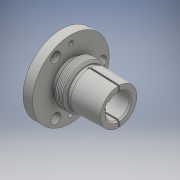
# Autodesk Inventor part: Spannhylsa_2015_HT1
Saved by Autodesk Inventor 2016 (Build 200138000, 138)
## iProperties
Created: 2015-09-08
Part Number: Spannhylsa_2015_HT1
Material: Generic
Document SubType Name: Modeling
Designer: hesaon
Density: 1 g/cm^3
Appearance: Default
Author: hesaon
Title: Spannhylsa_2015_HT1
Autodesk Inventor part; units mm, degrees
ref_plane "YZ Plane" through (0, 0, 0) normal (1, 0, 0) x (0, 1, 0)
ref_plane "XY Plane" through (0, 0, 0) normal (0, 0, 1) x (1, 0, 0)
sketch "Sketch1" plane through (0, 0, 0) normal (0, 0, 1) x (1, 0, 0)
  line L0 (0, 0) -> (60, 0)
  line L1 (0, 0) -> (0, 12.5) construction
  line L2 (0, 40) -> (10, 40)
  line L3 (10, 40) -> (10, 19)
  line L4 (10, 19) -> (14, 19)
  line L5 (0, 12.5) -> (60, 12.5)
  line L6 (60, 12.5) -> (60, 18.9524)
  line L7 (30, 20) -> (30, 19)
  line L8 (30, 19) -> (26, 19)
  line L9 (26, 19) -> (26, 19.9019)
  line L10 (14, 19.9019) -> (14, 19)
  line L11 (15.5, 22.5) -> (14, 19.9019)
  line L12 (15.5, 22.5) -> (24.5, 22.5)
  line L13 (24.5, 22.5) -> (26, 19.9019)
  line L14 (30, 20) -> (60, 18.9524)
  line L15 (30, 20) -> (60.0183, 20) construction
  arc A0 (0, 18.75) -> (0, 21.25) centre (0, 20) ccw
  line L16 (0, 12.5) -> (0, 18.75)
  line L17 (0, 21.25) -> (0, 40)
  dimension "d0" = 60
  dimension "d1" = 12.5
  dimension "d2" = 27.5
  dimension "d3" = 10
  dimension "d4" = 21
  dimension "d5" = 4
  dimension "d9" = 4
  dimension "d11" = 1
  dimension "d20" = 1.5
  dimension "d21" = 60
  dimension "d22" = 1.5
  dimension "d23" = 60
  dimension "d25" = 0.9019
  dimension "d26" = 0.9019
  dimension "d28" = 60
  dimension "d29" = 2
  dimension "d30" = 7.5
  dimension "d31" = 9
  dimension "d32" = 2.5
  dimension "d33" = 40
  constraints: 36 end point, 5 horizontal, 5 vertical, 4 perpendicular, 2 point on circle, 1 centre point, 1 equal length
  measures "d0" distance of L0.start L0.end
  measures "d1" distance of L0.start L1.end
  measures "d2" distance of L1.end L2.start
  measures "d3" distance of L2.start L2.end
  measures "d4" distance of L2.end L3.end
  measures "d5" distance of L3.end L4.end
  measures "d9" distance of L7.end L8.end
  measures "d11" distance of L7.start L7.end
  measures "d20" horizontal distance of L12.end L9.end
  measures "d21" angle of L13 L12
  measures "d22" horizontal distance of L11.start L10.start
  measures "d23" angle of L12 L11
  measures "d25" distance of L10.start L4.end
  measures "d26" distance of L8.end L9.end
  measures "d28" distance of L5.end L1.end
  measures "d29" angle of L14 L15
  measures "d30" vertical distance of L5.end L15.end
  measures "d31" distance of L11.start L12.end
  measures "d32" diameter of A0
  measures "d33" diameter of A0.centre L0
revolve "Revolution1" add sketch "Sketch1" angle 360 about axis through (0, 0, 0) along (1, 0, 0)
sketch "Sketch2" plane through (10, 0, 0) normal (1, 0, 0) x (0, 0, -1)
  point P0 (0, 0)
  point P1 (0, 32)
hole "Hole1" at (10, 32, 0) direction (-1, 0, 0) diameter 10.5 end through all
pattern_circular "Circular Pattern1" count 3 over 360 about axis through (30, 0, 0) along (1, 0, 0) of "Hole1"
sketch "Sketch3" plane through (10, 0, 0) normal (1, 0, 0) x (0, 0, -1)
  point P0 (0, 0)
  point P1 (0, 0)
  point P2 (32, 0)
  constraints: 1 coincident
hole "Hole2" at (10, 0, 0) at (10, 0, -32) direction (-1, 0, 0) diameter 5 end through all
pattern_circular "Circular Pattern2" count 2 over 360 about axis through (30, 0, 0) along (1, 0, 0) of "Hole2"
sketch "Sketch4" plane through (60, 0, 0) normal (1, 0, 0) x (0, 0, -1)
  line L0 (-62.0461, 0.75) -> (63.0717, 0.75)
  line L1 (63.0717, 0.75) -> (63.0717, -0.75)
  line L2 (63.0717, -0.75) -> (-62.0461, -0.75)
  line L3 (-62.0461, -0.75) -> (-62.0461, 0.75)
  point P0 (0, 0)
  dimension "d55" = 1.5
  dimension "d56" = 0.75
  constraints: 8 end point, 2 parallel, 1 horizontal, 1 perpendicular
  measures "d55" distance of L0.end L1.end
  measures "d56" distance from line of L0 point (0, 0)
extrude "Extrusion1" cut sketch "Sketch4" against normal blind 32
sketch "Sketch5" plane through (60, 0, 0) normal (1, 0, 0) x (0, 0, -1)
  line L0 (0, 0) -> (-26.5, -45.8993)
  line L1 (0, 0) -> (53, 0) construction
  line L2 (-2.1416, -9.7648) -> (-5.1902, -14.9339)
  line L3 (-5.1902, -14.9339) -> (-10.3584, -11.8858)
  line L4 (-10.3584, -11.8858) -> (-7.3098, -6.7168)
  line L5 (-7.3098, -6.7168) -> (-2.1416, -9.7648)
  circle A0 centre (0, 0) radius 12.5 projected
  line L6 (-2.1416, -9.7648) -> (-10.3584, -11.8858) construction
  line L7 (-5.1902, -14.9339) -> (-7.3098, -6.7168) construction
  point P0 (-6.25, -10.8253)
  dimension "d59" = 53
  dimension "d60" = 120
  dimension "d61" = 6
  dimension "d62" = 15.5
  constraints: 16 end point, 2 midpoint, 2 parallel, 1 equal length, 1 horizontal, 1 perpendicular, 1 point on line, 2 other
  measures "d59" distance of L0.start L0.end
  measures "d60" angle of L0 L1
  measures "d61" distance between parallel lines of L4 L2
  measures "d62" distance from line of L3 L0.start
extrude "Extrusion2" cut sketch "Sketch5" against normal through all contours L5 L2 A0 L0 | L0 A0 L4 L5 | A0 L2 L3 L0 | L0 L3 L4 A0
chamfer "Chamfer1" distance 1.5 angle 45 3 edges at (60, -5.24, 11.3487) (60, 12.5, 0) (60, -10.2103, -7.2111)
thread "Thread1" size "M45x1.5" class "6g" standard "ISO Metric profile" full length
ref_plane "Work Plane1" through (0, 17.5, 0) normal (0, 1, 0) x (-1, 0, 0)
sketch "Sketch6" plane through (0, 17.5, 0) normal (0, 1, 0) x (-1, 0, 0)
  line L0 (-38, 0) -> (-50, 0) construction
  line L1 (-38, 4) -> (-50, 4)
  line L2 (-50, -4) -> (-38, -4)
  arc A0 (-38, -4) -> (-38, 4) centre (-38, 0) ccw
  arc A1 (-50, 4) -> (-50, -4) centre (-50, 0) ccw
  point P0 (0, 0)
  point P1 (-44, 0)
  dimension "d71" = 8
  dimension "d72" = 38
  dimension "d73" = 50
  constraints: 8 end point, 4 point on circle, 4 tangent, 2 centre point, 1 horizontal, 1 midpoint, 1 parallel
  measures "d71" distance between parallel lines of L2 L1
  measures "d72" distance of L0.start point (0, 0)
  measures "d73" distance of L0.end point (0, 0)
extrude "Extrusion3" cut sketch "Sketch6" along normal blind 26.5
equation "\"d56\" = 0.5 * d55"
equation "\"d22\" = d20"
equation "\"d23\" = d21"
equation "\"d26\" = d25"
body "Solid1"
